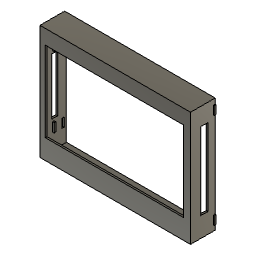
Pantry case v4 (Autodesk Fusion 360 design; units mm, degrees)
Autodesk Fusion 360 part; units mm, degrees
sketch "Sketch1" plane through (0, 0, 0) normal (0, 1, 0) x (1, 0, 0)
  line L0 (0, -130) -> (171, -130)
  line L1 (171, -130) -> (171, 0)
  line L2 (171, 0) -> (0, 0)
  line L3 (0, 0) -> (0, -130)
  line L4 (6, -113.5) -> (163, -113.5)
  line L5 (163, -113.5) -> (163, -22.5)
  line L6 (163, -22.5) -> (6, -22.5)
  line L7 (6, -22.5) -> (6, -113.5)
  line L8 (2, -128) -> (169, -128)
  line L9 (169, -128) -> (169, -2)
  line L10 (169, -2) -> (2, -2)
  line L11 (2, -2) -> (2, -128)
  circle A0 centre (6, -8.1) radius 3
  circle A1 centre (164, -8.1) radius 3
  circle A2 centre (6, -123) radius 3
  circle A3 centre (164, -123) radius 3
  dimension "d1" = 171
  dimension "d2" = 130
  dimension "d3" = 157
  dimension "d4" = 91
  dimension "d6" = 16.5
  dimension "d7" = 167
  dimension "d8" = 126
  dimension "d9" = 2
  dimension "d10" = 2
  dimension "d15" = 6
  dimension "d17" = 14.4
  dimension "d18" = 6
  dimension "d19" = 158
  dimension "d20" = 6
  dimension "d21" = 6
  dimension "d22" = 158
  dimension "d25" = 7
  dimension "d37" = 14.4
  dimension "d39" = 7
  dimension "d40" = 114.9
  constraint horizontal L0
  constraint vertical L1
  constraint horizontal L2
  constraint vertical L3
  constraint coincident L2.end L3.start
  constraint horizontal L4
  constraint vertical L5
  constraint horizontal L6
  constraint vertical L7
  constraint horizontal L8
  constraint vertical L9
  constraint horizontal L10
  constraint vertical L11
  measures "d1" distance of L0.start L0.end
  measures "d2" distance of L0.start L2.end
  measures "d3" distance of L4.start L4.end
  measures "d4" distance of L4.start L6.end
  measures "d6" distance of L0 L4
  measures "d7" distance of L8.start L8.end
  measures "d8" distance of L8.start L10.end
  measures "d9" distance of L0 L8
  measures "d10" distance of L3 L11
  measures "d15" diameter of A0
  measures "d17" distance of L6 A0.centre
  measures "d18" diameter of A1
  measures "d19" distance of A0.centre A1.centre
  measures "d20" diameter of A2
  measures "d21" diameter of A3
  measures "d22" distance of A3.centre A2.centre
  measures "d25" distance of L1 A3.centre
  measures "d37" distance of L6 A1.centre
  measures "d39" distance of L1 A1.centre
  measures "d40" distance of A1.centre A3.centre
extrude "Extrude1" add sketch "Sketch1" along normal blind 28 contours L0 L1 L2 L3
extrude "Extrude2" add sketch "Sketch1" along normal blind 2 contours L8 L9 L10 L11 | A0 | A1 | A2 | A3
extrude "Extrude4" add sketch "Sketch1" along normal blind 10.7 contours A3
extrude "Extrude5" add sketch "Sketch1" along normal blind 10.7 contours A2
extrude "Extrude6" add sketch "Sketch1" along normal blind 10.7 contours A0
extrude "Extrude7" add sketch "Sketch1" along normal blind 10.7 contours A1
fillet "Fillet1" radius 2 1 edges at (161.203, 2, 121.9152)
fillet "Fillet2" radius 2 1 edges at (3.203, 2, 121.9152)
fillet "Fillet3" radius 2 1 edges at (3.203, 2, 7.0152)
fillet "Fillet4" radius 2 1 edges at (161.203, 2, 7.0152)
sketch "Right - Buttons" plane through (0, 0, 0) normal (1, 0, 0) x (0, 1, 0)
  line L0 (11.5, 97) -> (18.2, 97)
  line L1 (18.2, 97) -> (18.2, 33)
  line L2 (18.2, 33) -> (11.5, 33)
  line L3 (11.5, 33) -> (11.5, 97)
  line L4 (0, 0) -> (28, 0)
  line L5 (14.2, 110) -> (12.2, 110)
  line L6 (12.2, 110) -> (12.2, 100)
  line L7 (12.2, 100) -> (14.2, 100)
  line L8 (14.2, 100) -> (14.2, 110)
  line L9 (0, 130) -> (28, 130)
  line L10 (14.2, 30) -> (12.2, 30)
  line L11 (12.2, 30) -> (12.2, 20)
  line L12 (12.2, 20) -> (14.2, 20)
  line L13 (14.2, 20) -> (14.2, 30)
  line L14 (23, 112) -> (25.5, 112)
  line L15 (25.5, 112) -> (25.5, 102)
  line L16 (25.5, 102) -> (23, 102)
  line L17 (23, 102) -> (23, 112)
  line L18 (28, 0) -> (28, 130)
  line L19 (23, 28) -> (25.5, 28)
  line L20 (25.5, 28) -> (25.5, 18)
  line L21 (25.5, 18) -> (23, 18)
  line L22 (23, 18) -> (23, 28)
  dimension "d49" = 6.7
  dimension "d50" = 64
  dimension "d51" = 33
  dimension "d52" = 11.5
  dimension "d73" = 2
  dimension "d74" = 10
  dimension "d75" = 12.2
  dimension "d76" = 20
  dimension "d77" = 2
  dimension "d78" = 10
  dimension "d79" = 12.2
  dimension "d80" = 20
  dimension "d91" = 2.5
  dimension "d92" = 10
  dimension "d93" = 2.5
  dimension "d94" = 18
  dimension "d95" = 2.5
  dimension "d96" = 10
  dimension "d97" = 2.5
  dimension "d98" = 18
  constraint horizontal L0
  constraint vertical L1
  constraint horizontal L2
  constraint vertical L3
  constraint horizontal L5
  constraint vertical L6
  constraint horizontal L7
  constraint vertical L8
  constraint horizontal L10
  constraint vertical L11
  constraint horizontal L12
  constraint vertical L13
  constraint horizontal L14
  constraint vertical L15
  constraint horizontal L16
  constraint vertical L17
  constraint horizontal L19
  constraint vertical L20
  constraint horizontal L21
  constraint vertical L22
  measures "d49" distance of L0.start L0.end
  measures "d50" distance of L0.start L2.end
  measures "d51" distance of L2 L4
  measures "d52" distance of L4.start L3
  measures "d73" distance of L5.start L5.end
  measures "d74" distance of L5.start L7.end
  measures "d75" distance of L6 L4.start
  measures "d76" distance of L5 L9
  measures "d77" distance of L10.start L10.end
  measures "d78" distance of L10.start L12.end
  measures "d79" distance of L4.start L11
  measures "d80" distance of L4 L12
  measures "d91" distance of L14.start L14.end
  measures "d92" distance of L14.start L16.end
  measures "d93" distance of L15 L18
  measures "d94" distance of L9 L14
  measures "d95" distance of L19.start L19.end
  measures "d96" distance of L19.start L21.end
  measures "d97" distance of L18 L20
  measures "d98" distance of L4 L21
extrude "Extrude8" cut sketch "Right - Buttons" along normal blind 10 contours L0 L1 L2 L3
sketch "Left - HDMI" plane through (171, 0, 0) normal (1, 0, 0) x (0, 1, 0)
  line L0 (0, 130) -> (0, 0)
  line L1 (0, 0) -> (28, 0)
  line L2 (28, 0) -> (28, 130)
  line L3 (28, 130) -> (0, 130)
  line L4 (11.5, 110) -> (19.8, 110)
  line L5 (19.8, 110) -> (19.8, 22.5)
  line L6 (19.8, 22.5) -> (11.5, 22.5)
  line L7 (11.5, 22.5) -> (11.5, 110)
  line L8 (12.2, 124) -> (14.2, 124)
  line L9 (14.2, 124) -> (14.2, 114)
  line L10 (14.2, 114) -> (12.2, 114)
  line L11 (12.2, 114) -> (12.2, 124)
  line L12 (12.2, 16) -> (14.2, 16)
  line L13 (14.2, 16) -> (14.2, 6)
  line L14 (14.2, 6) -> (12.2, 6)
  line L15 (12.2, 6) -> (12.2, 16)
  line L16 (26, 124) -> (28, 124)
  line L17 (28, 124) -> (28, 114)
  line L18 (28, 114) -> (26, 114)
  line L19 (26, 114) -> (26, 124)
  line L20 (26, 16) -> (28, 16)
  line L21 (28, 16) -> (28, 6)
  line L22 (28, 6) -> (26, 6)
  line L23 (26, 6) -> (26, 16)
  dimension "d55" = 8.3
  dimension "d56" = 87.5
  dimension "d57" = 22.5
  dimension "d58" = 11.5
  dimension "d61" = 2
  dimension "d62" = 10
  dimension "d63" = 12.2
  dimension "d64" = 6
  dimension "d65" = 2
  dimension "d66" = 10
  dimension "d67" = 12.2
  dimension "d68" = 6
  dimension "d103" = 2
  dimension "d104" = 10
  dimension "d106" = 2
  dimension "d107" = 10
  constraint horizontal L4
  constraint vertical L5
  constraint horizontal L6
  constraint vertical L7
  constraint horizontal L8
  constraint vertical L9
  constraint horizontal L10
  constraint vertical L11
  constraint horizontal L12
  constraint vertical L13
  constraint horizontal L14
  constraint vertical L15
  constraint horizontal L16
  constraint vertical L17
  constraint horizontal L18
  constraint vertical L19
  constraint collinear L2 L17
  constraint collinear L8 L16
  constraint horizontal L20
  constraint vertical L21
  constraint horizontal L22
  constraint vertical L23
  constraint collinear L2 L21
  constraint collinear L12 L20
  measures "d55" distance of L4.start L4.end
  measures "d56" distance of L4.start L6.end
  measures "d57" distance of L1 L6
  measures "d58" distance of L0.end L7
  measures "d61" distance of L8.start L8.end
  measures "d62" distance of L8.start L10.end
  measures "d63" distance of L0.end L11
  measures "d64" distance of L3 L8
  measures "d65" distance of L12.start L12.end
  measures "d66" distance of L12.start L14.end
  measures "d67" distance of L0.end L15
  measures "d68" distance of L1 L14
  measures "d103" distance of L16.start L16.end
  measures "d104" distance of L16.start L18.end
  measures "d106" distance of L20.start L20.end
  measures "d107" distance of L20.start L22.end
extrude "Extrude9" cut sketch "Left - HDMI" against normal blind 5 contours L4 L5 L6 L7
extrude "Extrude10" add sketch "Left - HDMI" against normal blind 4.5 contours L8 L9 L10 L11
extrude "Extrude11" add sketch "Left - HDMI" against normal blind 4.5 contours L12 L13 L14 L15
extrude "Extrude12" add sketch "Right - Buttons" along normal blind 4 contours L5 L6 L7 L8
extrude "Extrude13" add sketch "Right - Buttons" along normal blind 4 contours L10 L11 L12 L13
extrude "Extrude14" cut sketch "Right - Buttons" along normal blind 3 contours L14 L15 L16 L17
extrude "Extrude15" cut sketch "Right - Buttons" along normal blind 3 contours L19 L20 L21 L22
extrude "Extrude16" add sketch "Left - HDMI" along normal blind 1 contours L2 L16 L17 L18 L19
extrude "Extrude17" add sketch "Left - HDMI" along normal blind 1 contours L2 L20 L21 L22 L23
